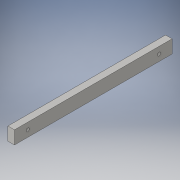
# Autodesk Inventor part: arm3
Saved by Autodesk Inventor 2016 (Build 200138000, 138)
## iProperties
Created: 2016-01-18
Part Number: arm3
Material: Generic
Document SubType Name: Modeling
Designer: Thariq
Density: 1 g/cm^3
Appearance: Default
Author: Thariq
Autodesk Inventor part; units mm, degrees
ref_plane "YZ Plane" through (0, 0, 0) normal (1, 0, 0) x (0, 1, 0)
ref_plane "XZ Plane" through (0, 0, 0) normal (0, 1, 0) x (-1, 0, 0)
ref_plane "XY Plane" through (0, 0, 0) normal (0, 0, 1) x (1, 0, 0)
sketch "Sketch1" plane through (0, 0, 0) normal (0, 1, 0) x (-1, 0, 0)
  line L0 (0, 0) -> (-12.7, 0)
  line L1 (-12.7, 0) -> (-12.7, 304.8)
  line L2 (-12.7, 304.8) -> (0, 304.8)
  line L3 (0, 304.8) -> (0, 0)
  dimension "d0" = 304.8
  dimension "d1" = 12.7
  constraints: 8 end point, 2 parallel, 1 horizontal, 1 perpendicular
  measures "d0" distance between parallel lines of L0 L2
  measures "d1" distance between parallel lines of L3 L1
extrude "Extrusion1" add sketch "Sketch1" along normal blind 25.4
sketch "Sketch2" plane through (12.7, 0, 304.8) normal (1, 0, 0) x (0, 0, -1)
  circle A0 centre (279.4, 12.7) radius 3.175
  line L0 (304.8, 0) -> (304.8, 25.4) projected
  line L1 (0, 25.4) -> (304.8, 25.4) projected
  circle A1 centre (25.4, 12.7) radius 3.175
  line L2 (0, 0) -> (0, 25.4) projected
  line L3 (304.8, 0) -> (0, 0) projected
  dimension "d4" = 6.35
  dimension "d5" = 25.4
  dimension "d6" = 12.7
  dimension "d7" = 6.35
  dimension "d8" = 25.4
  dimension "d9" = 12.7
  constraints: 2 centre point
  measures "d4" diameter of A0
  measures "d5" distance from line of L0 A0.centre
  measures "d6" distance from line of L1 A0.centre
  measures "d7" diameter of A1
  measures "d8" distance from line of L2 A1.centre
  measures "d9" distance from line of L3 A1.centre
extrude "Extrusion2" cut sketch "Sketch2" against normal through all contours A0 | A1
body "Solid1"
